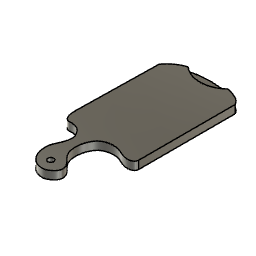
Cutting Board v15 (Autodesk Fusion 360 design; units mm, degrees)
Autodesk Fusion 360 part; units mm, degrees
sketch "Sketch1" plane through (0, 0, 0) normal (0, 0, 1) x (1, 0, 0)
  line L0 (65.2561, 92.8515) -> (-175.6842, 92.8608)
  line L1 (-167.4743, -89.0901) -> (37.3652, -93)
  spline S0 degree 5 poles (-175.6842, 92.8608) (-176.8835, 92.2501) (-179.2219, 90.8749) (-182.5491, 88.3508) (-186.6232, 84.0589) (-191.1042, 77.1514) (-194.965, 68.7444) (-198.2007, 58.9554) (-200.8143, 48.0111) (-202.8121, 36.2108) (-204.2003, 23.8931) (-204.9807, 11.4032) (-205.1483, -0.9393) (-204.6882, -12.8734) (-203.5736, -24.2276) (-201.7704, -34.8988) (-199.2419, -44.8371) (-195.9536, -54.0291) (-191.8791, -62.484) (-187.0076, -70.2185) (-181.3424, -77.2495) (-176.1823, -82.324) (-171.9634, -85.8251) (-168.9964, -88.0242) (-167.4743, -89.0901) knots 0 0 0 0 0 0 0.05 0.1 0.15 0.2 0.25 0.3 0.35 0.4 0.45 0.5 0.55 0.6 0.65 0.7 0.75 0.8 0.85 0.9 0.95 1 1 1 1 1 1
  spline S1 degree 5 poles (64.4631, 92.8515) (64.9542, 92.8668) (65.9169, 92.8506) (67.3029, 92.6862) (69.0343, 92.1867) (70.9997, 91.0973) (72.7516, 89.5497) (74.2605, 87.5575) (75.4807, 85.1439) (76.3645, 82.3461) (76.873, 79.2194) (76.9878, 75.8413) (76.7241, 72.3172) (76.126, 68.7676) (75.2567, 65.31) (74.1898, 62.0419) (73.0001, 59.0237) (71.7548, 56.2606) (70.5056, 53.6899) (69.2934, 51.2092) (68.1513, 48.7018) (67.1087, 46.0616) (66.1953, 43.2222) (65.4418, 40.1687) (64.8773, 36.9221) (64.5255, 33.5289) (64.4026, 30.05) (64.5139, 26.5487) (64.8515, 23.0805) (65.4002, 19.6932) (66.1418, 16.4267) (67.0607, 13.3122) (68.1483, 10.3723) (69.4097, 7.6203) (70.8609, 5.0611) (72.5209, 2.6928) (74.404, 0.5091) (76.5128, -1.4996) (78.8293, -3.344) (81.3202, -5.0352) (83.9475, -6.5835) (86.6779, -7.9979) (89.4918, -9.2855) (92.3943, -10.4503) (95.4091, -11.4927) (98.5676, -12.409) (101.8993, -13.1904) (105.4225, -13.8227) (109.1329, -14.2852) (113.0002, -14.5516) (116.9769, -14.5932) (121.0037, -14.3816) (125.0159, -13.8921) (128.95, -13.106) (132.7502, -12.0142) (136.3741, -10.6194) (139.7933, -8.9363) (142.9931, -6.9911) (145.9727, -4.8213) (148.7455, -2.4755) (151.3386, -0.013) (153.7938, 2.4962) (156.1622, 4.9762) (158.4983, 7.3513) (160.8545, 9.5517) (163.2758, 11.5187) (165.7929, 13.2112) (168.4195, 14.6078) (171.1545, 15.6951) (173.9837, 16.4586) (176.8817, 16.8751) (179.8137, 16.8991) (182.7376, 16.4685) (185.6072, 15.5289) (188.374, 14.055) (190.9905, 12.0694) (193.413, 9.6709) (195.6026, 7.018) (197.5269, 4.2855) (199.1605, 1.6285) (200.4861, -0.8526) (201.496, -3.1577) (202.1923, -5.3949) (202.5869, -7.7077) (202.7009, -10.2228) (202.5653, -12.9802) (202.2186, -15.9023) (201.6985, -18.8541) (201.0342, -21.6882) (200.24, -24.2908) (199.3045, -26.6401) (198.1964, -28.7993) (196.8801, -30.8651) (195.3269, -32.933) (193.5315, -35.0476) (191.5142, -37.1898) (189.3086, -39.3051) (186.9515, -41.3229) (184.4741, -43.1765) (181.8889, -44.8285) (179.1919, -46.2723) (176.3733, -47.5199) (173.4252, -48.5939) (170.3502, -49.5184) (167.1719, -50.3089) (163.9333, -50.9689) (160.6849, -51.4928) (157.4745, -51.8676) (154.3379, -52.0744) (151.287, -52.09) (148.3035, -51.8897) (145.3521, -51.4528) (142.3899, -50.7685) (139.3781, -49.8415) (136.2928, -48.6983) (133.1337, -47.3901) (129.9162, -45.9829) (126.6662, -44.5494) (123.4146, -43.1589) (120.1914, -41.8703) (117.0194, -40.7207) (113.9115, -39.7263) (110.8702, -38.8949) (107.8866, -38.2348) (104.9402, -37.7644) (101.9975, -37.5235) (99.0137, -37.5774) (95.9489, -37.995) (92.7809, -38.8323) (89.5185, -40.1141) (86.217, -41.8149) (82.9867, -43.8454) (79.9625, -46.0829) (77.2785, -48.3951) (75.0391, -50.6681) (73.2949, -52.8297) (72.0075, -54.8821) (71.0548, -56.9008) (70.2962, -58.9825) (69.6156, -61.2105) (68.9898, -63.6025) (68.4801, -66.11) (68.1641, -68.6568) (68.0908, -71.164) (68.2111, -73.5873) (68.3704, -75.9249) (68.3738, -78.1917) (68.0297, -80.4034) (67.2125, -82.5525) (65.8715, -84.6056) (64.0007, -86.5174) (61.6211, -88.2395) (58.7545, -89.7322) (55.4152, -90.9681) (51.6133, -91.9286) (47.3548, -92.6026) (43.5852, -92.9084) (40.5544, -93.0056) (38.4433, -93.0116) (37.3652, -93) knots 0 0 0 0 0 0 0.00645161 0.01290323 0.01935484 0.02580645 0.03225806 0.03870968 0.04516129 0.0516129 0.05806452 0.06451613 0.07096774 0.07741935 0.08387097 0.09032258 0.09677419 0.10322581 0.10967742 0.11612903 0.12258065 0.12903226 0.13548387 0.14193548 0.1483871 0.15483871 0.16129032 0.16774194 0.17419355 0.18064516 0.18709677 0.19354839 0.2 0.20645161 0.21290323 0.21935484 0.22580645 0.23225806 0.23870968 0.24516129 0.2516129 0.25806452 0.26451613 0.27096774 0.27741935 0.28387097 0.29032258 0.29677419 0.30322581 0.30967742 0.31612903 0.32258065 0.32903226 0.33548387 0.34193548 0.3483871 0.35483871 0.36129032 0.36774194 0.37419355 0.38064516 0.38709677 0.39354839 0.4 0.40645161 0.41290323 0.41935484 0.42580645 0.43225806 0.43870968 0.44516129 0.4516129 0.45806452 0.46451613 0.47096774 0.47741935 0.48387097 0.49032258 0.49677419 0.50322581 0.50967742 0.51612903 0.52258065 0.52903226 0.53548387 0.54193548 0.5483871 0.55483871 0.56129032 0.56774194 0.57419355 0.58064516 0.58709677 0.59354839 0.6 0.60645161 0.61290323 0.61935484 0.62580645 0.63225806 0.63870968 0.64516129 0.6516129 0.65806452 0.66451613 0.67096774 0.67741935 0.68387097 0.69032258 0.69677419 0.70322581 0.70967742 0.71612903 0.72258065 0.72903226 0.73548387 0.74193548 0.7483871 0.75483871 0.76129032 0.76774194 0.77419355 0.78064516 0.78709677 0.79354839 0.8 0.80645161 0.81290323 0.81935484 0.82580645 0.83225806 0.83870968 0.84516129 0.8516129 0.85806452 0.86451613 0.87096774 0.87741935 0.88387097 0.89032258 0.89677419 0.90322581 0.90967742 0.91612903 0.92258065 0.92903226 0.93548387 0.94193548 0.9483871 0.95483871 0.96129032 0.96774194 0.97419355 0.98064516 0.98709677 0.99354839 1 1 1 1 1 1
  circle A0 centre (174.0251, -17.3286) radius 7.5
  point P0 (-194.7795, 68.4746)
  point P1 (-205, 0)
  point P2 (-194.3178, -57.109)
  point P3 (72.1831, 89.9573)
  point P4 (76.8362, 78.4048)
  point P5 (73.1458, 59.4716)
  point P6 (67.5349, 47.0781)
  point P7 (64.4631, 30.4299)
  point P8 (67.5471, 12.0792)
  point P9 (75, 0)
  point P10 (87.2656, -8.2389)
  point P11 (103.9525, -13.5338)
  point P12 (128.8225, -13.0525)
  point P13 (149.0394, -2.1418)
  point P14 (162.5173, 10.8548)
  point P15 (175.5138, 16.631)
  point P16 (189.3127, 13.2616)
  point P17 (200, 0)
  point P18 (202.6301, -9.5225)
  point P19 (200.7047, -22.6796)
  point P20 (196, -32)
  point P21 (186, -42)
  point P22 (172, -49)
  point P23 (155, -52)
  point P24 (140, -50)
  point P25 (121.9231, -42.5755)
  point P26 (105.7175, -37.9224)
  point P27 (90, -40)
  point P28 (74.1085, -51.8817)
  point P29 (70, -60)
  point P30 (68.1502, -70.0463)
  point P31 (68.1718, -79.1584)
  point P32 (62.9013, -87.2409)
  dimension "d5" = 15
  constraint coincident L0 S1.start
  constraint coincident L1 S1.end
  constraint coincident S1 L1.end
  constraint coincident S1 L0.start
  measures "d5" diameter of A0
extrude "Extrude1" add sketch "Sketch1" along normal blind 20 contours L0 L1 S0 S1
sketch "Sketch2" plane through (0, 0, 20) normal (0, 0, 1) x (-1, 0, 0)
  circle A0 centre (-174.0251, 17.3286) radius 7.5
  spline S0 degree 5 poles (175.6842, -92.8608) (176.8835, -92.2501) (179.2219, -90.8749) (182.5491, -88.3508) (186.6232, -84.0589) (191.1042, -77.1514) (194.965, -68.7444) (198.2007, -58.9554) (200.8143, -48.0111) (202.8121, -36.2108) (204.2003, -23.8931) (204.9807, -11.4032) (205.1483, 0.9393) (204.6882, 12.8734) (203.5736, 24.2276) (201.7704, 34.8988) (199.2419, 44.8371) (195.9536, 54.0291) (191.8791, 62.484) (187.0076, 70.2185) (181.3424, 77.2495) (176.1823, 82.324) (171.9634, 85.8251) (168.9964, 88.0242) (167.4743, 89.0901) knots 0 0 0 0 0 0 0.05 0.1 0.15 0.2 0.25 0.3 0.35 0.4 0.45 0.5 0.55 0.6 0.65 0.7 0.75 0.8 0.85 0.9 0.95 1 1 1 1 1 1
  line L0 (167.4743, 89.0901) -> (-37.3652, 93)
  spline S1 degree 5 poles (-37.3652, 93) (-38.4433, 93.0116) (-40.5544, 93.0056) (-43.5852, 92.9084) (-47.3548, 92.6026) (-51.6133, 91.9286) (-55.4152, 90.9681) (-58.7545, 89.7322) (-61.6211, 88.2395) (-64.0007, 86.5174) (-65.8715, 84.6056) (-67.2125, 82.5525) (-68.0297, 80.4034) (-68.3738, 78.1917) (-68.3704, 75.9249) (-68.2111, 73.5873) (-68.0908, 71.164) (-68.1641, 68.6568) (-68.4801, 66.11) (-68.9898, 63.6025) (-69.6156, 61.2105) (-70.2962, 58.9825) (-71.0548, 56.9008) (-72.0075, 54.8821) (-73.2949, 52.8297) (-75.0391, 50.6681) (-77.2785, 48.3951) (-79.9625, 46.0829) (-82.9867, 43.8454) (-86.217, 41.8149) (-89.5185, 40.1141) (-92.7809, 38.8323) (-95.9489, 37.995) (-99.0137, 37.5774) (-101.9975, 37.5235) (-104.9402, 37.7644) (-107.8866, 38.2348) (-110.8702, 38.8949) (-113.9115, 39.7263) (-117.0194, 40.7207) (-120.1914, 41.8703) (-123.4146, 43.1589) (-126.6662, 44.5494) (-129.9162, 45.9829) (-133.1337, 47.3901) (-136.2928, 48.6983) (-139.3781, 49.8415) (-142.3899, 50.7685) (-145.3521, 51.4528) (-148.3035, 51.8897) (-151.287, 52.09) (-154.3379, 52.0744) (-157.4745, 51.8676) (-160.6849, 51.4928) (-163.9333, 50.9689) (-167.1719, 50.3089) (-170.3502, 49.5184) (-173.4252, 48.5939) (-176.3733, 47.5199) (-179.1919, 46.2723) (-181.8889, 44.8285) (-184.4741, 43.1765) (-186.9515, 41.3229) (-189.3086, 39.3051) (-191.5142, 37.1898) (-193.5315, 35.0476) (-195.3269, 32.933) (-196.8801, 30.8651) (-198.1964, 28.7993) (-199.3045, 26.6401) (-200.24, 24.2908) (-201.0342, 21.6882) (-201.6985, 18.8541) (-202.2186, 15.9023) (-202.5653, 12.9802) (-202.7009, 10.2228) (-202.5869, 7.7077) (-202.1923, 5.3949) (-201.496, 3.1577) (-200.4861, 0.8526) (-199.1605, -1.6285) (-197.5269, -4.2855) (-195.6026, -7.018) (-193.413, -9.6709) (-190.9905, -12.0694) (-188.374, -14.055) (-185.6072, -15.5289) (-182.7376, -16.4685) (-179.8137, -16.8991) (-176.8817, -16.8751) (-173.9837, -16.4586) (-171.1545, -15.6951) (-168.4195, -14.6078) (-165.7929, -13.2112) (-163.2758, -11.5187) (-160.8545, -9.5517) (-158.4983, -7.3513) (-156.1622, -4.9762) (-153.7938, -2.4962) (-151.3386, 0.013) (-148.7455, 2.4755) (-145.9727, 4.8213) (-142.9931, 6.9911) (-139.7933, 8.9363) (-136.3741, 10.6194) (-132.7502, 12.0142) (-128.95, 13.106) (-125.0159, 13.8921) (-121.0037, 14.3816) (-116.9769, 14.5932) (-113.0002, 14.5516) (-109.1329, 14.2852) (-105.4225, 13.8227) (-101.8993, 13.1904) (-98.5676, 12.409) (-95.4091, 11.4927) (-92.3943, 10.4503) (-89.4918, 9.2855) (-86.6779, 7.9979) (-83.9475, 6.5835) (-81.3202, 5.0352) (-78.8293, 3.344) (-76.5128, 1.4996) (-74.404, -0.5091) (-72.5209, -2.6928) (-70.8609, -5.0611) (-69.4097, -7.6203) (-68.1483, -10.3723) (-67.0607, -13.3122) (-66.1418, -16.4267) (-65.4002, -19.6932) (-64.8515, -23.0805) (-64.5139, -26.5487) (-64.4026, -30.05) (-64.5255, -33.5289) (-64.8773, -36.9221) (-65.4418, -40.1687) (-66.1953, -43.2222) (-67.1087, -46.0616) (-68.1513, -48.7018) (-69.2934, -51.2092) (-70.5056, -53.6899) (-71.7548, -56.2606) (-73.0001, -59.0237) (-74.1898, -62.0419) (-75.2567, -65.31) (-76.126, -68.7676) (-76.7241, -72.3172) (-76.9878, -75.8413) (-76.873, -79.2194) (-76.3645, -82.3461) (-75.4807, -85.1439) (-74.2605, -87.5575) (-72.7516, -89.5497) (-70.9997, -91.0973) (-69.1629, -92.1154) (-67.585, -92.602) (-66.3673, -92.7893) (-65.5779, -92.8412) (-65.2561, -92.8515) knots -1 -1 -1 -1 -1 -1 -0.99354839 -0.98709677 -0.98064516 -0.97419355 -0.96774194 -0.96129032 -0.95483871 -0.9483871 -0.94193548 -0.93548387 -0.92903226 -0.92258065 -0.91612903 -0.90967742 -0.90322581 -0.89677419 -0.89032258 -0.88387097 -0.87741935 -0.87096774 -0.86451613 -0.85806452 -0.8516129 -0.84516129 -0.83870968 -0.83225806 -0.82580645 -0.81935484 -0.81290323 -0.80645161 -0.8 -0.79354839 -0.78709677 -0.78064516 -0.77419355 -0.76774194 -0.76129032 -0.75483871 -0.7483871 -0.74193548 -0.73548387 -0.72903226 -0.72258065 -0.71612903 -0.70967742 -0.70322581 -0.69677419 -0.69032258 -0.68387097 -0.67741935 -0.67096774 -0.66451613 -0.65806452 -0.6516129 -0.64516129 -0.63870968 -0.63225806 -0.62580645 -0.61935484 -0.61290323 -0.60645161 -0.6 -0.59354839 -0.58709677 -0.58064516 -0.57419355 -0.56774194 -0.56129032 -0.55483871 -0.5483871 -0.54193548 -0.53548387 -0.52903226 -0.52258065 -0.51612903 -0.50967742 -0.50322581 -0.49677419 -0.49032258 -0.48387097 -0.47741935 -0.47096774 -0.46451613 -0.45806452 -0.4516129 -0.44516129 -0.43870968 -0.43225806 -0.42580645 -0.41935484 -0.41290323 -0.40645161 -0.4 -0.39354839 -0.38709677 -0.38064516 -0.37419355 -0.36774194 -0.36129032 -0.35483871 -0.3483871 -0.34193548 -0.33548387 -0.32903226 -0.32258065 -0.31612903 -0.30967742 -0.30322581 -0.29677419 -0.29032258 -0.28387097 -0.27741935 -0.27096774 -0.26451613 -0.25806452 -0.2516129 -0.24516129 -0.23870968 -0.23225806 -0.22580645 -0.21935484 -0.21290323 -0.20645161 -0.2 -0.19354839 -0.18709677 -0.18064516 -0.17419355 -0.16774194 -0.16129032 -0.15483871 -0.1483871 -0.14193548 -0.13548387 -0.12903226 -0.12258065 -0.11612903 -0.10967742 -0.10322581 -0.09677419 -0.09032258 -0.08387097 -0.07741935 -0.07096774 -0.06451613 -0.05806452 -0.0516129 -0.04516129 -0.03870968 -0.03225806 -0.02580645 -0.01935484 -0.01290323 -0.00645161 -0.00211087 -0.00211087 -0.00211087 -0.00211087 -0.00211087 -0.00211087
  line L1 (-65.2561, -92.8515) -> (175.6842, -92.8608)
  arc A1 (198.2244, 47.248) -> (200.1592, -50.1758) centre (251.463, -0.4258) ccw
  constraint coincident S0 A1.end
  constraint coincident S0 A1.start
extrude "Extrude2" cut sketch "Sketch2" against normal blind 10 contours S0 A1
move_body "Move1" bodies 1 to x (0, -1, 0) y (1, 0, 0) z (0, 0, 1) at (107.9324, 208.8165, 0)
